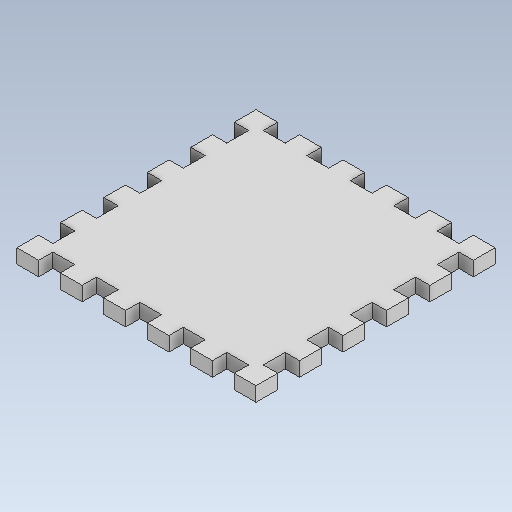
# Autodesk Inventor part: base
Saved by Autodesk Inventor 2020 (Build 240168000, 168)
## iProperties
Created: 2020-03-06
Part Number: base
Material: Generic
Document SubType Name: Modeling
Designer: udvarhelyi
Density: 1 g/cm^3
Appearance: Default
Author: udvarhelyi
Autodesk Inventor part; units mm, degrees
ref_plane "YZ Plane" through (0, 0, 0) normal (1, 0, 0) x (0, 1, 0)
ref_plane "XZ Plane" through (0, 0, 0) normal (0, 1, 0) x (-1, 0, 0)
ref_plane "XY Plane" through (0, 0, 0) normal (0, 0, 1) x (1, 0, 0)
sketch "Sketch1" plane through (0, 0, 0) normal (0, 1, 0) x (-1, 0, 0)
  line L0 (20.4545, 25) -> (20.4545, 22)
  line L1 (15.9091, 22) -> (15.9091, 25)
  line L2 (11.3636, 25) -> (11.3636, 22)
  line L3 (6.8182, 22) -> (6.8182, 25)
  line L4 (2.2727, 25) -> (2.2727, 22)
  line L5 (-2.2727, 22) -> (-2.2727, 25)
  line L6 (-6.8182, 25) -> (-6.8182, 22)
  line L7 (-11.3636, 22) -> (-11.3636, 25)
  line L8 (-15.9091, 25) -> (-15.9091, 22)
  line L9 (-20.4545, 22) -> (-20.4545, 25)
  line L10 (-25, 20.4545) -> (-22, 20.4545)
  line L11 (-22, 15.9091) -> (-25, 15.9091)
  line L12 (-25, 11.3636) -> (-22, 11.3636)
  line L13 (-22, 6.8182) -> (-25, 6.8182)
  line L14 (-25, 2.2727) -> (-22, 2.2727)
  line L15 (-22, -2.2727) -> (-25, -2.2727)
  line L16 (-22, -6.8182) -> (-25, -6.8182)
  line L17 (-25, -11.3636) -> (-22, -11.3636)
  line L18 (-22, -15.9091) -> (-25, -15.9091)
  line L19 (-25, -20.4545) -> (-22, -20.4545)
  line L20 (-20.4545, -25) -> (-20.4545, -22)
  line L21 (-15.9091, -22) -> (-15.9091, -25)
  line L22 (-11.3636, -25) -> (-11.3636, -22)
  line L23 (-6.8182, -22) -> (-6.8182, -25)
  line L24 (-2.2727, -22) -> (-2.2727, -25)
  line L25 (2.2727, -25) -> (2.2727, -22)
  line L26 (20.4545, -22) -> (20.4545, -25)
  line L27 (15.9091, -25) -> (15.9091, -22)
  line L28 (11.3636, -22) -> (11.3636, -25)
  line L29 (6.8182, -25) -> (6.8182, -22)
  line L30 (22, -20.4545) -> (25, -20.4545)
  line L31 (25, -15.9091) -> (22, -15.9091)
  line L32 (25, -11.3636) -> (22, -11.3636)
  line L33 (25, -2.2727) -> (22, -2.2727)
  line L34 (25, 2.2727) -> (22, 2.2727)
  line L35 (25, 20.4545) -> (22, 20.4545)
  line L36 (22, 15.9091) -> (25, 15.9091)
  line L37 (25, 11.3636) -> (22, 11.3636)
  line L38 (22, 6.8182) -> (25, 6.8182)
  line L39 (15.9091, -22) -> (20.4545, -22)
  line L40 (6.8182, -22) -> (11.3636, -22)
  line L41 (-2.2727, -22) -> (2.2727, -22)
  line L42 (22, -20.4545) -> (22, -15.9091)
  line L43 (22, -2.2727) -> (22, 2.2727)
  line L44 (22, 6.8182) -> (22, 11.3636)
  line L45 (22, 15.9091) -> (22, 20.4545)
  line L46 (20.4545, 22) -> (15.9091, 22)
  line L47 (11.3636, 22) -> (6.8182, 22)
  line L48 (2.2727, 22) -> (-2.2727, 22)
  line L49 (-6.8182, 22) -> (-11.3636, 22)
  line L50 (-15.9091, 22) -> (-20.4545, 22)
  line L51 (-22, 20.4545) -> (-22, 15.9091)
  line L52 (-22, 11.3636) -> (-22, 6.8182)
  line L53 (-22, 2.2727) -> (-22, -2.2727)
  line L54 (-25, 6.8182) -> (-25, 2.2727)
  line L55 (-25, 25) -> (-25, 20.4545)
  line L56 (-25, 15.9091) -> (-25, 11.3636)
  line L57 (-20.4545, -22) -> (-15.9091, -22)
  line L58 (-11.3636, -22) -> (-6.8182, -22)
  line L59 (-22, -6.8182) -> (-22, -11.3636)
  line L60 (-22, -15.9091) -> (-22, -20.4545)
  line L61 (-25, -2.2727) -> (-25, -6.8182)
  line L62 (-25, -11.3636) -> (-25, -15.9091)
  line L63 (-25, -20.4545) -> (-25, -25)
  line L64 (-25, -25) -> (-20.4545, -25)
  line L65 (-15.9091, -25) -> (-11.3636, -25)
  line L66 (-6.8182, -25) -> (-2.2727, -25)
  line L67 (2.2727, -25) -> (6.8182, -25)
  line L68 (11.3636, -25) -> (15.9091, -25)
  line L69 (20.4545, -25) -> (25, -25)
  line L70 (25, -25) -> (25, -20.4545)
  line L71 (25, 2.2727) -> (25, 6.8182)
  line L72 (25, 11.3636) -> (25, 15.9091)
  line L73 (25, 20.4545) -> (25, 25)
  line L74 (25, 25) -> (20.4545, 25)
  line L75 (15.9091, 25) -> (11.3636, 25)
  line L76 (6.8182, 25) -> (2.2727, 25)
  line L77 (-2.2727, 25) -> (-6.8182, 25)
  line L78 (-11.3636, 25) -> (-15.9091, 25)
  line L79 (-20.4545, 25) -> (-25, 25)
  line L80 (22, -11.3636) -> (22, -6.8182)
  line L81 (22, -6.8182) -> (25, -6.8182)
  line L82 (25, -15.9091) -> (25, -11.3636)
  line L83 (25, -6.8182) -> (25, -2.2727)
  point P0 (0, 0)
  dimension "d1" = 50
  dimension "d3" = 50
  dimension "d5" = 25
  dimension "d6" = 25
  dimension "d7" = 3
  dimension "d8" = 3
  dimension "d9" = 3
  dimension "d10" = 3
  dimension "d15" = 4.5454
  constraints: 249 perpendicular, 168 end point, 121 parallel, 56 collinear, 20 equal length, 6 horizontal, 1 vertical
  measures "d1" distance of L63.end L69.end
  measures "d3" distance of L69.end L73.end
  measures "d5" horizontal distance of L69.end point (0, 0)
  measures "d6" horizontal distance of L69.end point (0, 0)
  measures "d7" distance of L26.start L26.end
  measures "d8" distance of L30.start L30.end
  measures "d9" distance of L19.start L19.end
  measures "d10" distance of L9.start L9.end
  measures "d15" distance of L28.end L27.start
extrude "Extrusion1" add sketch "Sketch1" along normal blind 3
equation "\"d1\" = wt"
equation "\"d3\" = lt"
equation "\"d5\" = 0.5 * lt"
equation "\"d6\" = 0.5 * wt"
equation "\"d7\" = tt"
equation "\"d8\" = tt"
equation "\"d9\" = tt"
equation "\"d10\" = tt"
equation "\"d13\" = tt"
equation "\"wt\" = 50"
equation "\"tt\" = 3"
equation "\"tol\" = 0"
equation "\"tiroir\" = 25.4"
equation "\"nHoles\" = 101.6"
equation "\"shelfH\" = 35"
equation "\"d0\" = 0.5 * wt"
equation "\"d2\" = 0.5 * lt"
equation "\"lt\" = 50"
equation "\"d4\" = tt"
body "Solid1"
